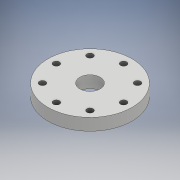
# Autodesk Inventor part: Nose Hub
Saved by Autodesk Inventor 2019 (Build 230136000, 136)
## iProperties
Created: 2017-06-23
Part Number: Nose Hub
Material: Generic
Document SubType Name: Modeling
Designer: t_crawk
Density: 1 g/cm^3
Appearance: Default
Author: t_crawk
Autodesk Inventor part; units mm, degrees
ref_plane "YZ Plane" through (0, 0, 0) normal (1, 0, 0) x (0, 1, 0)
ref_plane "XZ Plane" through (0, 0, 0) normal (0, 1, 0) x (-1, 0, 0)
ref_plane "XY Plane" through (0, 0, 0) normal (0, 0, 1) x (1, 0, 0)
sketch "Sketch1" plane through (0, 0, 0) normal (0, 0, 1) x (1, 0, 0)
  circle A0 centre (0, 0) radius 8.5
  circle A1 centre (0, 0) radius 35
  dimension "d0" = 17
  dimension "d1" = 70
  constraints: 2 centre point, 2 coincident
  measures "d0" diameter of A0
  measures "d1" diameter of A1
extrude "Extrusion1" add sketch "Sketch1" along normal blind 10
sketch "Sketch2" plane through (0, 0, 10) normal (0, 0, 1) x (1, 0, 0)
  circle A0 centre (0, 28) radius 2.2143
  point P0 (0, 0)
  dimension "d4" = 28
  constraints: 1 centre point
  measures "d4" distance of A0.centre point (0, 0)
hole "Hole1" at (0, 28, 10) direction (0, 0, -1) diameter 5.2 end through all
thread "Thread1" size "M5.5x0.5" class "6H" standard "ANSI Metric M Profile" full length
pattern_circular "Circular Pattern1" count 8 over 360 about axis through (0, 0, 0) along (0, 0, 1) of "Hole1"
body "Solid1"
